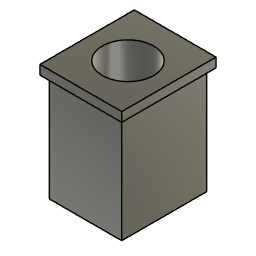
strut-pole-mount v1 (Autodesk Fusion 360 design; units mm, degrees)
Autodesk Fusion 360 part; units mm, degrees
sketch "Sketch1" plane through (0, 0, 0) normal (0, 0, 1) x (1, 0, 0)
  line L0 (15.55, 18.25) -> (-15.55, 18.25)
  line L1 (-15.55, 18.25) -> (-15.55, -18.25)
  line L2 (-15.55, -18.25) -> (15.55, -18.25)
  line L3 (15.55, -18.25) -> (15.55, 18.25)
  line L4 (15.55, 18.25) -> (-15.55, -18.25) construction
  line L5 (-15.55, 18.25) -> (15.55, -18.25) construction
  dimension "d1" = 31.1
  dimension "d2" = 36.5
  constraint horizontal L0
  constraint perpendicular L0 L1
  constraint parallel L0 L2
  constraint parallel L1 L3
  constraint coincident L4 origin
  constraint coincident L5 origin
  measures "d1" distance of L1.end L2.end
  measures "d2" distance of L0.end L1.end
extrude "Extrude1" add sketch "Sketch1" along normal blind 50
sketch "Sketch2" plane through (0, 0, 50) normal (0, 0, 1) x (-1, 0, 0)
  line L0 (-15.55, 18.25) -> (-15.55, -18.25)
  line L1 (-15.55, -18.25) -> (15.55, -18.25)
  line L2 (15.55, -18.25) -> (15.55, 18.25)
  line L3 (15.55, 18.25) -> (-15.55, 18.25)
  circle A0 centre (0, 0) radius 11
  dimension "d5" = 22
  constraint coincident A0.centre origin
  measures "d5" diameter of A0
extrude "Extrude2" cut sketch "Sketch2" against normal blind 16 contours A0
extrude "Extrude3" cut 1 faces at (-2.9076, 1.5312, 34) along direction (0, 0, -1) blind 69.898
sketch "Sketch3" plane through (0, 0, 50) normal (0, 0, 1) x (-1, 0, 0)
  circle A0 centre (0, 0) radius 11
  line L0 (-15.55, 18.25) -> (-15.55, -18.25)
  line L1 (-15.55, -18.25) -> (15.55, -18.25)
  line L2 (15.55, -18.25) -> (15.55, 18.25)
  line L3 (15.55, 18.25) -> (-15.55, 18.25)
  line L4 (-17.55, -20.25) -> (17.55, -20.25)
  line L5 (17.55, -20.25) -> (17.55, 20.25)
  line L6 (17.55, 20.25) -> (-17.55, 20.25)
  line L7 (-17.55, 20.25) -> (-17.55, -20.25)
  dimension "d10" = 2
extrude "Extrude4" add sketch "Sketch3" against normal blind 4 contours L0 L1 L2 L3 | L4 L5 L6 L7
